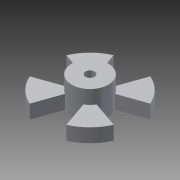
# Autodesk Inventor part: helice encodeur
Saved by Autodesk Inventor 2014 SP2 (Build 180246200, 246)
## iProperties
Created: 2015-03-17
Part Number: helice encodeur
Material: Plastique ABS
Document SubType Name: Modeling
Designer: sd
Density: 1.06 g/cm^3
Appearance: Lisse - Blanc
Mass: 0.144859 g
Surface Area: 2.23053 cm^2
Volume: 0.136659 cm^3
Author: sd
Autodesk Inventor part; units mm, degrees
ref_plane "YZ Plane" through (0, 0, 0) normal (1, 0, 0) x (0, 1, 0)
ref_plane "XZ Plane" through (0, 0, 0) normal (0, 1, 0) x (-1, 0, 0)
ref_plane "XY Plane" through (0, 0, 0) normal (0, 0, 1) x (1, 0, 0)
sketch "Esquisse1" plane through (0, 0, 0) normal (0, 0, 1) x (1, 0, 0)
  circle A0 centre (0, 0) radius 5
  dimension "d0" = 10
  constraints: 1 centre point, 1 coincident
  measures "d0" diameter of A0
extrude "Extrusion1" add sketch "Esquisse1" along normal blind 1.5
sketch "Esquisse2" plane through (0, 0, 1.5) normal (0, 0, 1) x (1, 0, 0)
  circle A0 centre (0, 0) radius 5 projected
  circle A1 centre (0, 0) radius 2
  dimension "d3" = 4
  constraints: 1 centre point, 1 coincident
  measures "d3" diameter of A1
extrude "Extrusion2" add sketch "Esquisse2" along normal blind 1.5 contours A1
sketch "Esquisse3" plane through (0, 0, 1.5) normal (0, 0, 1) x (1, 0, 0)
  circle A0 centre (0, 0) radius 2 projected
  circle A1 centre (0, 0) radius 5 projected
  line L0 (-2, 4.5826) -> (-1, 1.7321)
  line L1 (1, 1.7321) -> (2, 4.5826)
  arc A2 (1, 1.7321) -> (-1, 1.7321) centre (0, 0) ccw
  arc A3 (2, 4.5826) -> (-2, 4.5826) centre (0, 0) ccw
  constraints: 8 point on circle, 4 end point, 2 centre point, 2 concentric
extrude "Extrusion3" cut sketch "Esquisse3" against normal through all contours A0 L0 A1 L1 picked at (1.2132, 3.7931)
pattern_circular "Réseau circulaire1" count 4 over 360 about axis through (0, 0, 1.5) along (0, 0, 1) of "Extrusion3"
sketch "Esquisse4" plane through (0, 0, 3) normal (0, 0, 1) x (1, 0, 0)
  circle A0 centre (0, 0) radius 2 projected
  circle A1 centre (0, 0) radius 0.5
  dimension "d11" = 1
  constraints: 1 centre point, 1 coincident
  measures "d11" diameter of A1
extrude "Extrusion4" cut sketch "Esquisse4" against normal through all contours A1
